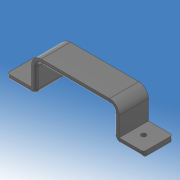
# Autodesk Inventor part: NASA-20-EBOX-LID-HANDLE-01
Saved by Autodesk Inventor 2020 (Build 240168000, 168)
## iProperties
Created: 2019-10-09
Part Number: NASA-20-EBOX-LID-HANDLE-01
Material: ABS Plastic
Document SubType Name: Modeling
Designer: mpark
Density: 1.06 g/cm^3
Appearance: Smooth - Black
Author: mpark
Autodesk Inventor part; units mm, degrees
ref_plane "YZ Plane" through (0, 0, 0) normal (1, 0, 0) x (0, 1, 0)
ref_plane "XZ Plane" through (0, 0, 0) normal (0, 1, 0) x (-1, 0, 0)
ref_plane "XY Plane" through (0, 0, 0) normal (0, 0, 1) x (1, 0, 0)
sketch "Sketch1" plane through (0, 0, 0) normal (0, 0, 1) x (1, 0, 0)
  line L0 (-88.9, 0) -> (-57.15, 0)
  line L1 (-50.8, 6.35) -> (-50.8, 31.75)
  line L2 (-44.45, 38.1) -> (44.45, 38.1)
  line L3 (50.8, 31.75) -> (50.8, 6.35)
  line L4 (57.15, 0) -> (88.9, 0)
  arc A0 (-44.45, 38.1) -> (-50.8, 31.75) centre (-44.45, 31.75) ccw
  arc A1 (50.8, 31.75) -> (44.45, 38.1) centre (44.45, 31.75) ccw
  arc A2 (-57.15, 0) -> (-50.8, 6.35) centre (-57.15, 6.35) ccw
  arc A3 (50.8, 6.35) -> (57.15, 0) centre (57.15, 6.35) ccw
  point P0 (0, 0)
  point P1 (-50.8, 0)
  point P2 (-50.8, 38.1)
  point P3 (50.8, 38.1)
  point P4 (50.8, 0)
  point P5 (0, 38.1)
  dimension "d0" = 38.1
  dimension "d1" = 38.1
  dimension "d2" = 38.1
  dimension "d3" = 101.6
  dimension "d4" = 6.35
  dimension "d5" = 6.35
  dimension "d6" = 6.35
  constraints: 10 end point, 10 point on line, 8 point on circle, 8 tangent, 4 centre point, 3 perpendicular, 1 equal radius, 1 horizontal, 1 horizontal alignment, 1 midpoint, 1 vertical alignment
  measures "d0" distance between parallel lines of L4 L2
  measures "d1" distance of L0.start point (-50.8, 0)
  measures "d2" distance of point (50.8, 0) L4.end
  measures "d3" distance of point (-50.8, 38.1) point (50.8, 38.1)
  measures "d4" radius of A0
  measures "d5" radius of A1
  measures "d6" radius of A2
surface extrude "ExtrusionSrf1" sketch "Sketch1" along normal blind 38.1 shown no curves L0 A2 L1 A0 L2 A1 L3 A3 L4
thicken "Thicken1" operation new thickness 6.35 both sides no extend neighbours no toward (0, 1, 0) faces at (-78.3167, 0, 12.7) (-51.6507, 3.175, 25.4) (-50.8, 14.8167, 12.7) (-49.6966, 35.3271, 25.4) (-14.8167, 38.1, 12.7) (48.0271, 36.9966, 25.4) (50.8, 23.2833, 12.7) (53.5729, 1.1034, 25.4) (67.7333, 0, 12.7)
fillet "Fillet1" radius 3.175 22 edges at (-88.9, 3.175, 38.1) (-88.9, 3.175, 0) (88.9, 3.175, 38.1) (88.9, 3.175, 0) (48.9401, 36.2401, 38.1) (0, 38.1, 38.1) (-48.9401, 36.2401, 38.1) (-50.8, 19.05, 38.1) (-52.6599, 1.8599, 38.1) (-73.025, 0, 38.1) (52.6599, 1.8599, 38.1) (73.025, 0, 38.1) (50.8, 19.05, 38.1) (-48.9401, 36.2401, 0) (0, 38.1, 0) (48.9401, 36.2401, 0) (50.8, 19.05, 0) (52.6599, 1.8599, 0) (73.025, 0, 0) (-52.6599, 1.8599, 0) (-73.025, 0, 0) (-50.8, 19.05, 0)
sketch "Sketch2" plane through (-57.15, 6.35, 38.1) normal (0, 1, 0) x (1, 0, 0)
  arc A0 (-28.575, 38.1) -> (-31.75, 34.925) centre (-28.575, 34.925) ccw projected
  line L0 (-31.75, 34.925) -> (-31.75, 3.175) projected
  arc A1 (-31.75, 3.175) -> (-28.575, 0) centre (-28.575, 3.175) ccw projected
  line L1 (0, 0) -> (-28.575, 0) projected
  line L2 (0, 38.1) -> (0, 0) projected
  line L3 (-28.575, 38.1) -> (0, 38.1) projected
  arc A2 (146.05, 34.925) -> (142.875, 38.1) centre (142.875, 34.925) ccw projected
  line L4 (114.3, 38.1) -> (142.875, 38.1) projected
  line L5 (114.3, 38.1) -> (114.3, 0) projected
  line L6 (142.875, 0) -> (114.3, 0) projected
  arc A3 (142.875, 0) -> (146.05, 3.175) centre (142.875, 3.175) ccw projected
  line L7 (146.05, 34.925) -> (146.05, 3.175) projected
  point P0 (57.15, 38.1)
  point P1 (-12.7, 19.05)
  point P2 (127, 19.05)
  dimension "d11" = 19.05
  dimension "d12" = 19.05
  dimension "d13" = 19.05
  constraints: 1 horizontal alignment
  measures "d11" distance from line of point (-12.7, 19.05) L0
  measures "d12" distance from line of L1 point (-12.7, 19.05)
  measures "d13" distance from line of L7 point (127, 19.05)
hole "Hole1" at (-69.85, 6.35, 19.05) at (69.85, 6.35, 19.05) direction (0, -1, 0) diameter 6.35 end through all
body "Solid1"
body "Srf1"
